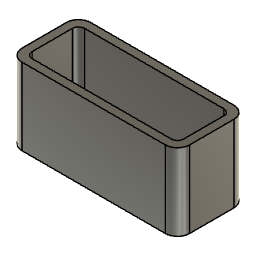
LarsBox v1 (Autodesk Fusion 360 design; units mm, degrees)
Autodesk Fusion 360 part; units mm, degrees
sketch "Sketch1" plane through (0, 0, 0) normal (0, 0, 1) x (1, 0, 0) in component "Box"
  line L0 (41.5, 17) -> (-41.5, 17)
  line L1 (-41.5, 17) -> (-41.5, -17)
  line L2 (-41.5, -17) -> (41.5, -17)
  line L3 (41.5, -17) -> (41.5, 17)
  line L4 (41.5, 17) -> (-41.5, -17) construction
  line L5 (-41.5, 17) -> (41.5, -17) construction
  dimension "d1" = 83
  dimension "d2" = 34
  constraint horizontal L0
  constraint perpendicular L0 L1
  constraint parallel L0 L2
  constraint parallel L1 L3
  constraint coincident L4 origin
  constraint coincident L5 origin
  measures "d1" distance of L1.end L2.end
  measures "d2" distance of L0.end L1.end
extrude "Extrude1" add sketch "Sketch1" along normal blind 38 in component "Box"
sketch "Sketch2" plane through (0, 0, 38) normal (0, 0, 1) x (-1, 0, 0) in component "Box"
  line L0 (-41.5, 17) -> (-41.5, -17)
  line L1 (-41.5, -17) -> (41.5, -17)
  line L2 (41.5, -17) -> (41.5, 17)
  line L3 (41.5, 17) -> (-41.5, 17)
  line L4 (-37.5, -13) -> (37.5, -13)
  line L5 (37.5, -13) -> (37.5, 13)
  line L6 (37.5, 13) -> (-37.5, 13)
  line L7 (-37.5, 13) -> (-37.5, -13)
  dimension "d5" = -4
extrude "Extrude2" cut sketch "Sketch2" against normal up to surface (34 mm away) contours L4 L5 L6 L7 in component "Box"
fillet "Fillet1" radius 3 4 edges at (37.5, 13, 21) (-37.5, 13, 21) (-37.5, -13, 21) (37.5, -13, 21) in component "Box"
fillet "Fillet2" radius 6 4 edges at (-41.5, 17, 19) (-41.5, -17, 19) (41.5, -17, 19) (41.5, 17, 19) in component "Box"
component "Box" placed x (1, 0, 0) y (0, 1, 0) z (0, 0, 1) at (0, 0, 0)
component "Lid" placed x (1, 0, 0) y (0, 1, 0) z (0, 0, 1) at (0, 0, 0)
